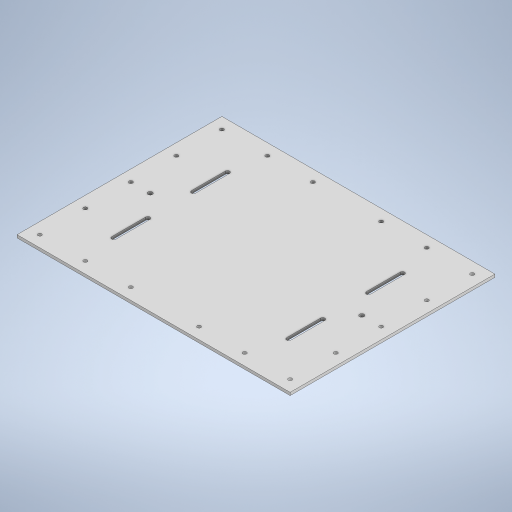
# Autodesk Inventor part: BatteryPlate
Saved by Autodesk Inventor 2023 (Build 270158000, 158)
## iProperties
Created: 2023-08-24
Part Number: BatteryPlate
Material: Generic
Document SubType Name: Modeling
Designer: jackc
Density: 1 g/cm^3
Appearance: Default
Author: jackc
Autodesk Inventor part; units mm, degrees
ref_plane "YZ Plane" through (0, 0, 0) normal (1, 0, 0) x (0, 1, 0)
ref_plane "XZ Plane" through (0, 0, 0) normal (0, 1, 0) x (-1, 0, 0)
ref_plane "XY Plane" through (0, 0, 0) normal (0, 0, 1) x (1, 0, 0)
sketch "Sketch1" plane through (0, 0, 0) normal (0, 1, 0) x (-1, 0, 0)
  line L0 (0, 0) -> (-304.8, 0)
  line L1 (-304.8, 0) -> (-304.8, -228.6)
  line L2 (-304.8, -228.6) -> (0, -228.6)
  line L3 (0, -228.6) -> (0, 0)
  line L4 (-12.7, -12.7) -> (-292.1, -12.7) construction
  line L5 (-292.1, -12.7) -> (-292.1, -215.9) construction
  line L6 (-292.1, -215.9) -> (-12.7, -215.9) construction
  line L7 (-12.7, -215.9) -> (-12.7, -12.7) construction
  circle A0 centre (-12.7, -12.7) radius 2.0701
  circle A1 centre (-12.7, -215.9) radius 2.0701
  circle A2 centre (-292.1, -12.7) radius 2.0701
  circle A3 centre (-292.1, -215.9) radius 2.0701
  circle A4 centre (-114.3, -12.7) radius 2.0701
  circle A5 centre (-63.5, -12.7) radius 2.0701
  circle A6 centre (-241.3, -12.7) radius 2.0701
  circle A7 centre (-12.7, -63.5) radius 2.0701
  circle A8 centre (-12.7, -114.3) radius 2.0701
  circle A9 centre (-12.7, -165.1) radius 2.0701
  circle A10 centre (-190.5, -215.9) radius 2.0701
  circle A11 centre (-63.5, -215.9) radius 2.0701
  circle A12 centre (-114.3, -215.9) radius 2.0701
  circle A13 centre (-292.1, -63.5) radius 2.0701
  circle A14 centre (-292.1, -114.3) radius 2.0701
  circle A15 centre (-292.1, -165.1) radius 2.0701
  circle A16 centre (-190.5, -12.7) radius 2.0701
  circle A17 centre (-241.3, -215.9) radius 2.0701
  point P0 (-12.7, -114.3)
  dimension "d0" = 304.8
  dimension "d1" = 228.6
  dimension "d2" = 12.7
  dimension "d3" = 12.7
  dimension "d4" = 12.7
  dimension "d5" = 12.7
  dimension "d6" = 4.1402
  dimension "d8" = 50.8
  dimension "d9" = 50.8
  dimension "d10" = 50.8
  dimension "d11" = 50.8
  dimension "d12" = 50.8
  dimension "d13" = 101.6
  dimension "d14" = 101.6
  constraints: 18 centre point, 17 equal radius, 16 end point, 12 point on line, 4 coincident, 4 parallel, 4 vertical alignment, 3 horizontal alignment, 3 midpoint, 2 horizontal, 2 perpendicular
  measures "d0" distance of L2.end L1.end
  measures "d1" distance of L1.end L0.end
  measures "d2" distance between parallel lines of L2 L6
  measures "d3" distance between parallel lines of L0 L4
  measures "d4" distance between parallel lines of L3 L7
  measures "d5" distance between parallel lines of L1 L5
  measures "d6" diameter of A0
  measures "d8" distance of L4.start A7.centre
  measures "d9" distance of A1.centre A9.centre
  measures "d10" distance of A7.centre A8.centre
  measures "d11" distance of L4.start A5.centre
  measures "d12" distance of L4.end A6.centre
  measures "d13" distance of L4.start A4.centre
  measures "d14" distance of L4.end A16.centre
extrude "Extrusion1" add sketch "Sketch1" along normal blind 3.175
sketch "Sketch2" plane through (0, 3.175, 0) normal (0, 1, 0) x (1, 0, 0)
  line L0 (57.15, 88.9) -> (57.15, 50.8) construction
  line L1 (54.7687, 88.9) -> (54.7687, 50.8)
  line L2 (59.5312, 50.8) -> (59.5312, 88.9)
  arc A0 (59.5312, 88.9) -> (54.7687, 88.9) centre (57.15, 88.9) ccw
  arc A1 (54.7687, 50.8) -> (59.5312, 50.8) centre (57.15, 50.8) ccw
  line L3 (0, 228.6) -> (0, 0) projected
  line L4 (304.8, 228.6) -> (0, 228.6) projected
  line L5 (57.15, 177.8) -> (57.15, 139.7) construction
  line L6 (54.7687, 177.8) -> (54.7687, 139.7)
  line L7 (59.5312, 139.7) -> (59.5312, 177.8)
  arc A2 (59.5312, 177.8) -> (54.7687, 177.8) centre (57.15, 177.8) ccw
  arc A3 (54.7687, 139.7) -> (59.5312, 139.7) centre (57.15, 139.7) ccw
  line L8 (252.4125, 177.8) -> (252.4125, 139.7) construction
  line L9 (250.0313, 177.8) -> (250.0313, 139.7)
  line L10 (254.7938, 139.7) -> (254.7938, 177.8)
  arc A4 (254.7938, 177.8) -> (250.0313, 177.8) centre (252.4125, 177.8) ccw
  arc A5 (250.0313, 139.7) -> (254.7938, 139.7) centre (252.4125, 139.7) ccw
  line L11 (252.4125, 88.9) -> (252.4125, 50.8) construction
  line L12 (250.0312, 88.9) -> (250.0312, 50.8)
  line L13 (254.7938, 50.8) -> (254.7938, 88.9)
  arc A6 (254.7938, 88.9) -> (250.0312, 88.9) centre (252.4125, 88.9) ccw
  arc A7 (250.0312, 50.8) -> (254.7938, 50.8) centre (252.4125, 50.8) ccw
  circle A8 centre (34.29, 114.3) radius 2.54
  circle A9 centre (270.51, 114.3) radius 2.54
  line L14 (304.8, 0) -> (304.8, 228.6) projected
  point P0 (57.15, 69.85)
  point P1 (0, 114.3)
  point P2 (152.4, 228.6)
  point P3 (0, 114.3)
  point P4 (57.15, 158.75)
  point P5 (252.4125, 158.75)
  point P6 (252.4125, 69.85)
  point P7 (250.0313, 158.75)
  point P8 (304.8, 114.3)
  dimension "d17" = 4.7625
  dimension "d18" = 38.1
  dimension "d19" = 25.4
  dimension "d20" = 50.8
  dimension "d21" = 190.5
  dimension "d22" = 95.25
  dimension "d25" = 5.08
  dimension "d26" = 34.29
  dimension "d27" = 34.29
  constraints: 32 end point, 16 point on circle, 16 tangent, 10 centre point, 10 midpoint, 5 parallel, 4 equal radius, 4 horizontal alignment, 3 equal length, 2 point on line, 2 vertical, 1 vertical alignment
  measures "d17" distance between parallel lines of L2 L1
  measures "d18" distance of L0.end L0.start
  measures "d19" vertical distance of point (0, 114.3) L0.start
  measures "d20" distance of L5.end L0.start
  measures "d21" distance from line of L7 point (250.031, 158.75)
  measures "d22" horizontal distance of point (152.4, 228.6) L5.start
  measures "d25" diameter of A8
  measures "d26" distance from line of L3 A8.centre
  measures "d27" distance from line of L14 A9.centre
extrude "Extrusion2" cut sketch "Sketch2" against normal blind 25.4
equation "\"d3\" = d2"
equation "\"d4\" = d2"
equation "\"d5\" = d2"
equation "\"d8\" = d9"
equation "\"d14\" = d13"
equation "\"d21\" = 2 * d22"
equation "\"d27\" = d26"
body "Solid1"
